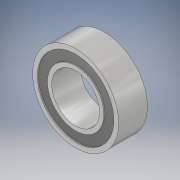
# Autodesk Inventor part: 9x5x3mm bearing
Saved by Autodesk Inventor 2017 (Build 210142000, 142)
## iProperties
Created: 2016-06-23
Part Number: 9x5x3mm bearing
Material: Generic
Document SubType Name: Modeling
Designer: Ben
Density: 1 g/cm^3
Appearance: Default
Author: Ben
Autodesk Inventor part; units mm, degrees
ref_plane "YZ Plane" through (0, 0, 0) normal (1, 0, 0) x (0, 1, 0)
ref_plane "XZ Plane" through (0, 0, 0) normal (0, 1, 0) x (-1, 0, 0)
ref_plane "XY Plane" through (0, 0, 0) normal (0, 0, 1) x (1, 0, 0)
sketch "Sketch1" plane through (0, 0, 0) normal (0, 0, 1) x (1, 0, 0)
  circle A0 centre (0, 0) radius 2.5
  circle A1 centre (0, 0) radius 4.5
  dimension "d0" = 9
  dimension "d1" = 5
  constraints: 2 centre point, 2 coincident
  measures "d0" diameter of A1
  measures "d1" diameter of A0
extrude "Extrusion1" add sketch "Sketch1" along normal blind 3
sketch "Sketch2" plane through (0, 0, 3) normal (0, 0, 1) x (1, 0, 0)
  circle A0 centre (0, 0) radius 2.5 projected
  circle A1 centre (0, 0) radius 4.5 projected
  circle A2 centre (0, 0) radius 2.95
  circle A3 centre (0, 0) radius 4
  dimension "d4" = 5.9
  dimension "d5" = 0.5
  constraints: 2 centre point, 2 coincident
  measures "d4" diameter of A2
  measures "d5" radial gap between concentric circles of A1 A3
extrude "Extrusion2" cut sketch "Sketch2" against normal blind 0.1 contours A3
sketch "Sketch3" plane through (0, 0, 0) normal (0, 0, -1) x (-1, 0, 0)
  circle A0 centre (0, 0) radius 4 projected
  circle A1 centre (0, 0) radius 2.95 projected
extrude "Extrusion3" cut sketch "Sketch3" against normal blind 0.1
body "Solid1"
